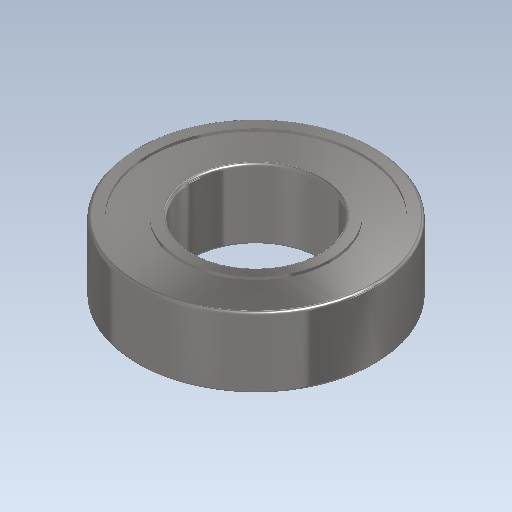
# Autodesk Inventor part: SUTB689ZZ
Saved by Autodesk Inventor 2021 (Build 250183000, 183)
## iProperties
Category: PARTsolutions
Company: MISUMI
Part Number: SUTB689ZZ
Material: ステンレス鋼
Catalog Web Link: www.cadenas.de
Description: SUTB_ _ _ ZZ-Prustro  Miniature Ball Bearings -Double Shield Type-
Vendor: MISUMI
Document SubType Name: Modeling
Designer: partserver
Manufacturer: MISUMI
Mass: 6.23037 g
Surface Area: 7.53656 cm^2
Volume: 0.778797 cm^3
Density: 8 g/cm^3
Appearance: 半つや出し
PSOL_IDENT_0: {$CADENAS_DATA\23d-libs\misumi\metric\12_bearing_holders\sutb692zz.prj},165 {VTYP=3D},{NB=SUTB689ZZ}
PSOL_IDENT_1: ,{LINA=SUTB689ZZ},{NN=SUTB_ _ _ ZZ},{DATE=09.09.2019 09:02:54},{GEOMDATE=25.05.2017 07:46:04},{VERSI
PSOL_IDENT_2: ON=},{LINEID=230},{WBVAR=},{WBNUMERIC=}  {NB=SUTB689ZZ},{LINA=SUTB689ZZ},{KT=DUMMY},{PN=SUTB689ZZ},{
PSOL_IDENT_3: TYPE=SUTB689ZZ},{BN=689ZZ},{DD=9},{D=17},{B=5.0},{RR=0.20},{B11=0.20},{D11=10.70},{D22=15.20},{CR=11
PSOL_IDENT_4: 30},{COR=530},{RRPPMM=36000},{DS=11.5},{DDHH=15.2},{R=0.2},{MASS=4.43}
NB: SUTB689ZZ
NN: SUTB_ _ _ ZZ
NT: Prustro  Miniature Ball Bearings -Double Shield Type-
NBSYN: $PN.
LINA: SUTB689ZZ
CATALOG: Misumi
PN: SUTB689ZZ
BN: 689ZZ
DD: 9
D: 17
B: 5
RR: 0.2
CR: 1130
COR: 530
RRPPMM: 36000
DS: 11.5
DDHH: 15.2
R: 0.2
MASS: 4.43
SUPPLIER: MISUMI
ARTICLENO: SUTB689ZZ
BOMINFO: SUTB689ZZ
CREATOR: CADENAS GmbH
d1: 0.000 mm
Title: SUTB689ZZ
Author: Cadenas PARTsolutions
Comments: Prustro  Miniature Ball Bearings -Double Shield Type-
Autodesk Inventor part; units mm, degrees
sketch "Sketch_1" plane through (0, 0, 0) normal (1, 0, 0) x (0, 0, -1)
  line L0 (5, 0) -> (0, 0)
  arc A0 (0, 4.7) -> (0.2, 4.5) centre (0.2, 4.7) ccw
  line L1 (0.2, 4.5) -> (4.8, 4.5)
  arc A1 (4.8, 4.5) -> (5, 4.7) centre (4.8, 4.7) ccw
  line L2 (5, 4.7) -> (5, 5.35)
  line L3 (5, 5.35) -> (4.8, 5.35)
  line L4 (4.8, 5.35) -> (4.8, 7.6)
  line L5 (4.8, 7.6) -> (5, 7.6)
  line L6 (5, 7.6) -> (5, 8.3)
  arc A2 (5, 8.3) -> (4.8, 8.5) centre (4.8, 8.3) ccw
  line L7 (4.8, 8.5) -> (0.2, 8.5)
  arc A3 (0.2, 8.5) -> (0, 8.3) centre (0.2, 8.3) ccw
  line L8 (0, 8.3) -> (0, 7.6)
  line L9 (0, 7.6) -> (0.2, 7.6)
  line L10 (0.2, 7.6) -> (0.2, 5.35)
  line L11 (0.2, 5.35) -> (0, 5.35)
  line L12 (0, 5.35) -> (0, 4.7)
  constraints: 26 end point, 8 point on circle, 4 centre point
revolve "Revolution1" add sketch "Sketch_1" angle 360 about axis through (0, 0, -5) along (0, 0, -1)
ref_plane "to_housing_XY" through (0, 0, 0) normal (0, 0, -1) x (1, 0, 0)
ref_plane "to_housing_YZ" through (0, 0, 0) normal (1, 0, 0) x (0, -1, 0)
ref_plane "to_housing_ZX" through (0, 0, 0) normal (0, -1, 0) x (0, 0, -1)
body "Solid1"
